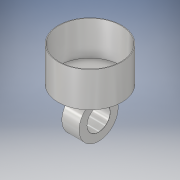
# Autodesk Inventor part: Conexion_inferior
Saved by Autodesk Inventor 2019 (Build 230136000, 136)
## iProperties
Created: 2019-09-23
Part Number: Conexion_inferior
Material: Genérico
Document SubType Name: Modeling
Designer: axelj
Density: 1 g/cm^3
Appearance: Aluminio - Pulido
Author: axelj
Autodesk Inventor part; units mm, degrees
ref_plane "YZ Plane" through (0, 0, 0) normal (1, 0, 0) x (0, 1, 0)
ref_plane "XZ Plane" through (0, 0, 0) normal (0, 1, 0) x (-1, 0, 0)
ref_plane "XY Plane" through (0, 0, 0) normal (0, 0, 1) x (1, 0, 0)
sketch "Boceto1" plane through (0, 0, 0) normal (0, 1, 0) x (-1, 0, 0)
  circle A0 centre (0, 0) radius 7
  dimension "d0" = 14
  constraints: 1 centre point, 1 coincident
  measures "d0" diameter of A0
extrude "Extrusión1" add sketch "Boceto1" along normal blind 7.7
sketch "Boceto2" plane through (0, 7.7, 0) normal (0, 1, 0) x (1, 0, 0)
  circle A0 centre (0, 0) radius 6.85
  dimension "d3" = 13.7
  constraints: 1 centre point, 1 coincident
  measures "d3" diameter of A0
extrude "Extrusión2" cut sketch "Boceto2" against normal blind 7.6
sketch "Boceto3" plane through (0, 0, 0) normal (0, -1, 0) x (1, 0, 0)
  circle A0 centre (0, 0) radius 2.5
  dimension "d6" = 5
  constraints: 1 centre point, 1 coincident
  measures "d6" diameter of A0
extrude "Extrusión3" add sketch "Boceto3" along normal blind 10
sketch "Boceto4" plane through (0, -10, 0) normal (0, -1, 0) x (1, 0, 0)
  arc A0 (-1.9, 1.6248) -> (-1.9, -1.6248) centre (0, 0) ccw
  arc A1 (1.9, -1.6248) -> (1.9, 1.6248) centre (0, 0) ccw
  circle A2 centre (0, 0) radius 2.5 projected
  line L0 (0, 0) -> (1.9, 0)
  line L1 (-1.9, 0) -> (-1.9, 1.6248)
  line L2 (-1.9, 0) -> (-1.9, -1.6248)
  line L3 (1.9, 0) -> (1.9, 1.6248)
  line L4 (1.9, 0) -> (1.9, -1.6248)
  point P0 (-1.6248, 1.9)
  point P1 (-1.6248, -1.9)
  point P2 (1.6248, -1.9)
  point P3 (1.6248, 1.9)
  constraints: 10 end point, 4 point on circle, 3 point on line, 2 centre point, 1 coincident, 1 horizontal, 1 parallel, 1 vertical, 5 other
extrude "Extrusión4" cut sketch "Boceto4" against normal blind 10 contours L1 L2 A0 | A1 L4 L3
sketch "Boceto6" plane through (1.9, -10, 1.6248) normal (1, 0, 0) x (0, 0, -1)
  line L0 (1.6248, 10) -> (1.6248, 8.6)
  circle A0 centre (1.6248, 4.3) radius 4.3
  dimension "d18" = 1.4
  dimension "d20" = 8.6
  constraints: 2 end point, 1 centre point, 1 vertical
  measures "d18" distance of L0.start L0.end
  measures "d20" diameter of A0
extrude "Extrusión5" add sketch "Boceto6" against normal blind 3.8
sketch "Boceto7" plane through (1.9, -10, 1.6248) normal (1, 0, 0) x (0, 0, -1)
  arc A0 (-0.8752, 0.8014) -> (4.1248, 0.8014) centre (1.6248, 4.3) ccw
  line L0 (3.2496, 0) -> (4.1248, 0) projected
  line L1 (-0.8752, 0) -> (0, 0) projected
  line L2 (4.1248, 0.8014) -> (4.1248, 0) projected
  line L3 (4.1248, 0.8014) -> (4.1248, 0)
  line L4 (-0.8752, 0.8014) -> (-0.8752, 0)
  line L5 (-0.8752, 0.8014) -> (-0.8752, 0) projected
  arc A1 (-0.8752, 0.8014) -> (4.1248, 0.8014) centre (1.6248, 4.3) ccw
  line L6 (-0.8752, 0) -> (1.6248, 0)
  line L7 (3.2496, 0) -> (0, 0) projected
  line L8 (1.6248, 0) -> (4.1248, 0)
  point P0 (1.6248, 10)
  constraints: 10 end point, 5 point on circle, 3 collinear, 2 centre point, 1 coincident, 1 midpoint
extrude "Extrusión6" cut sketch "Boceto7" against normal blind 3.8
sketch "Boceto8" plane through (-1.9, 0, -1.6248) normal (-1, 0, 0) x (0, 0, 1)
  circle A0 centre (1.6248, -5.7) radius 2.55
  point P0 (1.6248, 0)
  dimension "d28" = 5.1
  constraints: 1 centre point, 1 coincident
  measures "d28" diameter of A0
extrude "Extrusión7" cut sketch "Boceto8" against normal blind 3.8
fillet "Empalme1" radius 0.02 2 edges at (1.9, -5.7, -2.55) (-1.9, -5.7, -2.55)
